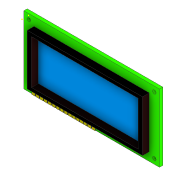
# Autodesk Inventor part: lcd display
Saved by Autodesk Inventor 2021 (Build 250183000, 183)
## iProperties
Created: 2021-06-25
Part Number: lcd display
Material: Generic
Document SubType Name: Modeling
Designer: Dell
Density: 1 g/cm^3
Appearance: Default
Author: Dell
Autodesk Inventor part; units mm, degrees
ref_plane "YZ Plane" through (0, 0, 0) normal (1, 0, 0) x (0, 1, 0)
ref_plane "XZ Plane" through (0, 0, 0) normal (0, 1, 0) x (-1, 0, 0)
sketch "Sketch2" plane through (0, 0, 0) normal (0, 0, 1) x (1, 0, 0)
  line L0 (-14.0665, 4.9582) -> (385.9335, 4.9582)
  line L1 (385.9335, 4.9582) -> (385.9335, -195.0418)
  line L2 (385.9335, -195.0418) -> (-14.0665, -195.0418)
  line L3 (-14.0665, -195.0418) -> (-14.0665, 4.9582)
  circle A0 centre (0.9335, -10.0418) radius 5
  circle A1 centre (370.9335, -10.0418) radius 5
  circle A2 centre (0.9335, -180.0418) radius 5
  circle A3 centre (370.9335, -180.0418) radius 5
  point P0 (0, 0)
  dimension "d3" = 400
  dimension "d4" = 200
  dimension "d5" = 10
  dimension "d6" = 10
  dimension "d7" = 10
  dimension "d8" = 10
  dimension "d9" = 15
  dimension "d10" = 15
  dimension "d11" = 15
  dimension "d12" = 15
  dimension "d13" = 15
  dimension "d14" = 15
  dimension "d15" = 15
  dimension "d16" = 15
  constraints: 8 end point, 4 centre point, 2 parallel, 1 horizontal, 1 perpendicular
  measures "d3" distance of L1.end L2.end
  measures "d4" distance of L0.end L1.end
  measures "d5" diameter of A0
  measures "d6" diameter of A1
  measures "d7" diameter of A2
  measures "d8" diameter of A3
  measures "d9" distance from line of L0 A0.centre
  measures "d10" distance from line of L3 A0.centre
  measures "d11" distance from line of L2 A2.centre
  measures "d12" distance from line of L3 A2.centre
  measures "d13" distance from line of L1 A1.centre
  measures "d14" distance from line of L0 A1.centre
  measures "d15" distance from line of L1 A3.centre
  measures "d16" distance from line of L2 A3.centre
extrude "Extrusion1" add sketch "Sketch2" along normal blind 10
sketch "Sketch3" plane through (0, 0, 10) normal (0, 0, 1) x (1, 0, 0)
  line L0 (15.9335, -20.0418) -> (355.9335, -20.0418)
  line L1 (355.9335, -20.0418) -> (355.9335, -170.0418)
  line L2 (355.9335, -170.0418) -> (15.9335, -170.0418)
  line L3 (15.9335, -170.0418) -> (15.9335, -20.0418)
  line L4 (385.9335, 4.9582) -> (-14.0665, 4.9582) projected
  line L5 (385.9335, -195.0418) -> (385.9335, 4.9582) projected
  point P0 (0, 0)
  dimension "d20" = 340
  dimension "d21" = 150
  dimension "d22" = 25
  dimension "d23" = 30
  constraints: 8 end point, 2 parallel, 1 horizontal, 1 perpendicular
  measures "d20" distance of L1.end L2.end
  measures "d21" distance of L0.end L1.end
  measures "d22" distance between parallel lines of L0 L4
  measures "d23" distance between parallel lines of L5 L1
extrude "Extrusion2" add sketch "Sketch3" along normal blind 20
sketch "Sketch4" plane through (0, 0, 30) normal (0, 0, 1) x (1, 0, 0)
  point P0 (0, 0)
sketch "Sketch5" plane through (0, 0, 30) normal (0, 0, 1) x (1, 0, 0)
  point P0 (0, 0)
sketch "Sketch6" plane through (0, 0, 30) normal (0, 0, 1) x (1, 0, 0)
  line L0 (-14.0665, -195.0418) -> (385.9335, -195.0418) projected
  line L1 (10.9169, -195.0418) -> (10.9169, -178.0418)
  line L2 (10.9169, -195.0418) -> (20.9169, -195.0418)
  line L3 (20.9169, -195.0418) -> (20.9169, -178.0418)
  arc A0 (20.9169, -178.0418) -> (10.9169, -178.0418) centre (15.9169, -178.0418) ccw
  line L4 (20.9169, -195.0418) -> (22.9169, -195.0418)
  line L5 (22.9169, -195.0418) -> (22.9169, -178.0418)
  line L6 (22.9169, -195.0418) -> (32.9169, -195.0418)
  line L7 (32.9169, -195.0418) -> (32.9169, -178.0418)
  arc A1 (32.9169, -178.0418) -> (22.9169, -178.0418) centre (27.9169, -178.0418) ccw
  line L8 (34.9169, -195.0418) -> (34.9169, -178.0418)
  line L9 (34.9169, -195.0418) -> (44.9169, -195.0418)
  line L10 (44.9169, -195.0418) -> (44.9169, -178.0418)
  arc A2 (44.9169, -178.0418) -> (34.9169, -178.0418) centre (39.9169, -178.0418) ccw
  line L11 (46.9169, -195.0418) -> (46.9169, -178.0418)
  line L12 (46.9169, -195.0418) -> (56.9169, -195.0418)
  line L13 (56.9169, -195.0418) -> (56.9169, -178.0418)
  arc A3 (56.9169, -178.0418) -> (46.9169, -178.0418) centre (51.9169, -178.0418) ccw
  line L14 (58.9169, -195.0418) -> (58.9169, -178.0418)
  line L15 (58.9169, -195.0418) -> (68.9169, -195.0418)
  line L16 (68.9169, -195.0418) -> (68.9169, -178.0418)
  arc A4 (68.9169, -178.0418) -> (58.9169, -178.0418) centre (63.9169, -178.0418) ccw
  line L17 (70.9169, -195.0418) -> (70.9169, -178.0418)
  line L18 (70.9169, -195.0418) -> (80.9169, -195.0418)
  line L19 (80.9169, -195.0418) -> (80.9169, -178.0418)
  arc A5 (80.9169, -178.0418) -> (70.9169, -178.0418) centre (75.9169, -178.0418) ccw
  line L20 (82.9169, -195.0418) -> (82.9169, -178.0418)
  line L21 (82.9169, -195.0418) -> (92.9169, -195.0418)
  line L22 (92.9169, -195.0418) -> (92.9169, -178.0418)
  arc A6 (92.9169, -178.0418) -> (82.9169, -178.0418) centre (87.9169, -178.0418) ccw
  line L23 (94.9169, -195.0418) -> (94.9169, -178.0418)
  line L24 (94.9169, -195.0418) -> (104.9169, -195.0418)
  line L25 (104.9169, -195.0418) -> (104.9169, -178.0418)
  arc A7 (104.9169, -178.0418) -> (94.9169, -178.0418) centre (99.9169, -178.0418) ccw
  line L26 (106.9169, -195.0418) -> (106.9169, -178.0418)
  line L27 (106.9169, -195.0418) -> (116.9169, -195.0418)
  line L28 (116.9169, -195.0418) -> (116.9169, -178.0418)
  arc A8 (116.9169, -178.0418) -> (106.9169, -178.0418) centre (111.9169, -178.0418) ccw
  line L29 (118.9169, -195.0418) -> (118.9169, -178.0418)
  line L30 (118.9169, -195.0418) -> (128.9169, -195.0418)
  line L31 (128.9169, -195.0418) -> (128.9169, -178.0418)
  arc A9 (128.9169, -178.0418) -> (118.9169, -178.0418) centre (123.9169, -178.0418) ccw
  line L32 (129.9169, -195.0418) -> (129.9169, -178.0418)
  line L33 (129.9169, -195.0418) -> (139.9169, -195.0418)
  line L34 (139.9169, -195.0418) -> (139.9169, -178.0418)
  arc A10 (139.9169, -178.0418) -> (129.9169, -178.0418) centre (134.9169, -178.0418) ccw
  line L35 (141.9169, -195.0418) -> (141.9169, -178.0418)
  line L36 (141.9169, -195.0418) -> (151.9169, -195.0418)
  line L37 (151.9169, -195.0418) -> (151.9169, -178.0418)
  arc A11 (151.9169, -178.0418) -> (141.9169, -178.0418) centre (146.9169, -178.0418) ccw
  line L38 (152.9169, -195.0418) -> (152.9169, -178.0418)
  line L39 (152.9169, -195.0418) -> (162.9169, -195.0418)
  line L40 (162.9169, -195.0418) -> (162.9169, -178.0418)
  arc A12 (162.9169, -178.0418) -> (152.9169, -178.0418) centre (157.9169, -178.0418) ccw
  line L41 (163.9169, -195.0418) -> (163.9169, -178.0418)
  line L42 (163.9169, -195.0418) -> (173.9169, -195.0418)
  line L43 (173.9169, -195.0418) -> (173.9169, -178.0418)
  arc A13 (173.9169, -178.0418) -> (163.9169, -178.0418) centre (168.9169, -178.0418) ccw
  line L44 (185.9169, -195.0418) -> (185.9169, -178.0418)
  line L45 (175.9169, -195.0418) -> (185.9169, -195.0418)
  line L46 (175.9169, -195.0418) -> (175.9169, -178.0418)
  arc A14 (185.9169, -178.0418) -> (175.9169, -178.0418) centre (180.9169, -178.0418) ccw
  line L47 (197.9169, -195.0418) -> (197.9169, -178.0418)
  line L48 (187.9169, -195.0418) -> (197.9169, -195.0418)
  line L49 (187.9169, -195.0418) -> (187.9169, -178.0418)
  arc A15 (197.9169, -178.0418) -> (187.9169, -178.0418) centre (192.9169, -178.0418) ccw
  line L50 (28.4335, -30.0418) -> (343.4335, -30.0418)
  line L51 (343.4335, -30.0418) -> (343.4335, -160.0418)
  line L52 (343.4335, -160.0418) -> (28.4335, -160.0418)
  line L53 (28.4335, -160.0418) -> (28.4335, -30.0418)
  line L54 (355.9335, -20.0418) -> (15.9335, -20.0418) projected
  line L55 (15.9335, -20.0418) -> (15.9335, -170.0418) projected
  point P0 (0, 0)
  dimension "d27" = 17
  dimension "d28" = 10
  dimension "d29" = 17
  dimension "d30" = 2
  dimension "d31" = 10
  dimension "d32" = 17
  dimension "d33" = 5
  dimension "d34" = 10
  dimension "d35" = 17
  dimension "d36" = 5
  dimension "d37" = 10
  dimension "d38" = 17
  dimension "d39" = 5
  dimension "d40" = 10
  dimension "d41" = 17
  dimension "d42" = 5
  dimension "d43" = 10
  dimension "d44" = 17
  dimension "d45" = 5
  dimension "d46" = 10
  dimension "d47" = 17
  dimension "d48" = 5
  dimension "d49" = 10
  dimension "d50" = 17
  dimension "d51" = 5
  dimension "d52" = 10
  dimension "d53" = 17
  dimension "d54" = 5
  dimension "d55" = 10
  dimension "d56" = 17
  dimension "d57" = 5
  dimension "d58" = 10
  dimension "d59" = 17
  dimension "d60" = 5
  dimension "d61" = 10
  dimension "d62" = 17
  dimension "d63" = 5
  dimension "d64" = 10
  dimension "d65" = 17
  dimension "d66" = 5
  dimension "d67" = 10
  dimension "d68" = 17
  dimension "d69" = 5
  dimension "d70" = 2
  dimension "d71" = 2
  dimension "d72" = 2
  dimension "d73" = 2
  dimension "d74" = 2
  dimension "d75" = 2
  dimension "d76" = 2
  dimension "d77" = 2
  dimension "d78" = 1
  dimension "d79" = 2
  dimension "d80" = 1
  dimension "d81" = 1
  dimension "d82" = 10
  dimension "d83" = 17
  dimension "d84" = 5
  dimension "d85" = 10
  dimension "d86" = 17
  dimension "d87" = 5
  dimension "d88" = 2
  dimension "d89" = 2
  dimension "d90" = 315
  constraints: 106 end point, 32 point on circle, 16 centre point, 3 vertical, 2 parallel, 2 perpendicular, 1 horizontal, 1 tangent, 5 other
  measures "d27" distance of L1.start L1.end
  measures "d28" distance of L1.start L2.end
  measures "d29" distance of L2.end L3.end
  measures "d30" distance of L2.end L4.end
  measures "d31" distance of L4.end L6.end
  measures "d32" distance of L6.end L7.end
  measures "d33" radius of A1
  measures "d34" distance of L9.start L10.start
  measures "d35" distance of L10.start L10.end
  measures "d36" radius of A2
  measures "d37" distance of L12.start L13.start
  measures "d38" distance of L13.start L13.end
  measures "d39" radius of A3
  measures "d40" distance of L15.start L16.start
  measures "d41" distance of L16.start L16.end
  measures "d42" radius of A4
  measures "d43" distance of L18.start L19.start
  measures "d44" distance of L19.start L19.end
  measures "d45" radius of A5
  measures "d46" distance of L21.start L22.start
  measures "d47" distance of L22.start L22.end
  measures "d48" radius of A6
  measures "d49" distance of L24.start L25.start
  measures "d50" distance of L25.start L25.end
  measures "d51" radius of A7
  measures "d52" distance of L27.start L28.start
  measures "d53" distance of L28.start L28.end
  measures "d54" radius of A8
  measures "d55" distance of L30.start L31.start
  measures "d56" distance of L31.start L31.end
  measures "d57" radius of A9
  measures "d58" distance of L33.start L34.start
  measures "d59" distance of L34.start L34.end
  measures "d60" radius of A10
  measures "d61" distance of L36.start L37.start
  measures "d62" distance of L37.start L37.end
  measures "d63" radius of A11
  measures "d64" distance of L39.start L40.start
  measures "d65" distance of L40.start L40.end
  measures "d66" radius of A12
  measures "d67" distance of L42.start L43.start
  measures "d68" distance of L43.start L43.end
  measures "d69" radius of A13
  measures "d70" distance between parallel lines of L8 L7
  measures "d71" distance between parallel lines of L11 L10
  measures "d72" distance between parallel lines of L14 L13
  measures "d73" distance between parallel lines of L17 L16
  measures "d74" distance between parallel lines of L20 L19
  measures "d75" distance between parallel lines of L23 L22
  measures "d76" distance between parallel lines of L26 L25
  measures "d77" distance between parallel lines of L29 L28
  measures "d78" distance from line of L31.start L32
  measures "d79" distance between parallel lines of L35 L34
  measures "d80" distance between parallel lines of L38 L37
  measures "d81" distance between parallel lines of L41 L40
  measures "d82" distance of L45.start L45.end
  measures "d83" distance of L45.end L44.end
  measures "d84" radius of A14
  measures "d85" distance of L48.start L48.end
  measures "d86" distance of L48.end L47.end
  measures "d87" radius of A15
  measures "d88" distance between parallel lines of L46 L43
  measures "d89" distance between parallel lines of L49 L44
  measures "d90" distance of L51.end L52.end
extrude "Extrusion3" add sketch "Sketch6" along normal blind 1 contours L1 A0 L3 L0 | L5 A1 L7 L0 | L8 A2 L10 L0 | L11 A3 L13 L0 | L14 A4 L16 L0 | L17 A5 L19 L0 | L20 A6 L22 L0 | L23 A7 L25 L0 | L26 A8 L28 L0 | L29 A9 L31 L0 | L32 A10 L34 L0 | L35 A11 L37 L0 | L38 A12 L40 L0 | L41 A13 L43 L0 | L46 A14 L44 L0 | L49 A15 L47 L0
sketch "Sketch7" plane through (0, 0, 30) normal (0, 0, 1) x (1, 0, 0)
  point P0 (0, 0)
sketch "Sketch8" plane through (0, 0, 30) normal (0, 0, 1) x (1, 0, 0)
  line L0 (28.4335, -30.0418) -> (343.4335, -30.0418)
  line L1 (343.4335, -30.0418) -> (343.4335, -160.0418)
  line L2 (343.4335, -160.0418) -> (28.4335, -160.0418)
  line L3 (28.4335, -160.0418) -> (28.4335, -30.0418)
  line L4 (355.9335, -20.0418) -> (15.9335, -20.0418) projected
  line L5 (15.9335, -20.0418) -> (15.9335, -170.0418) projected
  point P0 (0, 0)
  dimension "d96" = 315
  dimension "d97" = 130
  dimension "d98" = 10
  dimension "d99" = 12.5
  constraints: 8 end point, 2 parallel, 1 horizontal, 1 perpendicular
  measures "d96" distance of L1.end L2.end
  measures "d97" distance of L0.end L1.end
  measures "d98" distance between parallel lines of L0 L4
  measures "d99" distance between parallel lines of L5 L3
extrude "Extrusion4" cut sketch "Sketch8" against normal blind 20
sketch "Sketch9" plane through (0, 0, 10) normal (0, 0, 1) x (1, 0, 0)
  point P0 (0, 0)
sketch "Sketch10" plane through (0, 0, 10) normal (0, 0, 1) x (1, 0, 0)
  point P0 (0, 0)
sketch "Sketch11" plane through (0, 0, 10) normal (0, 0, 1) x (1, 0, 0)
  point P0 (0, 0)
sketch "Sketch12" plane through (0, 0, 10) normal (0, 0, 1) x (1, 0, 0)
  point P0 (0, 0)
ref_plane "Work Plane1" through (0, 0, 11) normal (0, 0, 1) x (1, 0, 0)
sketch "Sketch13" plane through (0, 0, 10) normal (0, 0, 1) x (1, 0, 0)
  point P0 (0, 0)
sketch "Sketch14" plane through (0, 0, 10) normal (0, 0, 1) x (1, 0, 0)
  point P0 (0, 0)
thicken "Thicken1" operation add thickness 20 both sides no extend neighbours no toward (0, 0, -1) faces at (14.2503, -183.7084, 31)
thicken "Thicken2" operation add thickness 20 both sides no extend neighbours no toward (0, 0, -1) faces at (26.2503, -183.7084, 31)
thicken "Thicken3" operation add thickness 20 both sides no extend neighbours no toward (0, 0, -1) faces at (41.5836, -183.7084, 31)
thicken "Thicken4" operation add thickness 20 both sides no extend neighbours no toward (0, 0, -1) faces at (53.5836, -183.7084, 31)
thicken "Thicken5" operation add thickness 20 both sides no extend neighbours no toward (0, 0, -1) faces at (65.5836, -183.7084, 31)
thicken "Thicken6" operation add thickness 20 both sides no extend neighbours no toward (0, 0, -1) faces at (74.2503, -189.3751, 31)
thicken "Thicken7" operation add thickness 20 both sides no extend neighbours no toward (0, 0, -1) faces at (86.2503, -189.3751, 31)
thicken "Thicken8" operation add thickness 20 both sides no extend neighbours no toward (0, 0, -1) faces at (98.2503, -189.3751, 31)
thicken "Thicken9" operation add thickness 20 both sides no extend neighbours no toward (0, 0, -1) faces at (110.2503, -189.3751, 31)
thicken "Thicken10" operation add thickness 20 both sides no extend neighbours no toward (0, 0, -1) faces at (122.2503, -189.3751, 31)
thicken "Thicken11" operation add thickness 20 both sides no extend neighbours no toward (0, 0, -1) faces at (133.2503, -183.7084, 31)
thicken "Thicken12" operation cut thickness 19 both sides no extend neighbours no toward (0, 0, -1) faces at (14.2503, -183.7084, 31)
thicken "Thicken13" operation add thickness 20 both sides no extend neighbours no toward (0, 0, -1) faces at (145.2503, -183.7084, 31)
thicken "Thicken14" operation add thickness 20 both sides no extend neighbours no toward (0, 0, -1) faces at (156.2503, -183.7084, 31)
thicken "Thicken15" operation add thickness 20 both sides no extend neighbours no toward (0, 0, -1) faces at (167.2503, -183.7084, 31)
thicken "Thicken16" operation add thickness 20 both sides no extend neighbours no toward (0, 0, -1) faces at (182.5836, -189.3751, 31)
thicken "Thicken17" operation add thickness 20 both sides no extend neighbours no toward (0, 0, -1) faces at (194.5836, -189.3751, 31)
thicken "Thicken18" operation cut thickness 19 both sides no extend neighbours no toward (0, 0, -1) faces at (26.2503, -183.7084, 31)
thicken "Thicken19" operation cut thickness 19 both sides no extend neighbours no toward (0, 0, -1) faces at (41.5836, -183.7084, 31)
thicken "Thicken20" operation cut thickness 19 both sides no extend neighbours no toward (0, 0, -1) faces at (53.5836, -183.7084, 31)
thicken "Thicken21" operation cut thickness 19 both sides no extend neighbours no toward (0, 0, -1) faces at (65.5836, -183.7084, 31)
thicken "Thicken22" operation cut thickness 19 both sides no extend neighbours no toward (0, 0, -1) faces at (74.2503, -189.3751, 31)
thicken "Thicken23" operation cut thickness 19 both sides no extend neighbours no toward (0, 0, -1) faces at (86.2503, -189.3751, 31)
thicken "Thicken24" operation cut thickness 19 both sides no extend neighbours no toward (0, 0, -1) faces at (98.2503, -189.3751, 31)
thicken "Thicken25" operation cut thickness 19 both sides no extend neighbours no toward (0, 0, -1) faces at (110.2503, -189.3751, 31)
thicken "Thicken26" operation cut thickness 19 both sides no extend neighbours no toward (0, 0, -1) faces at (122.2503, -189.3751, 31)
thicken "Thicken27" operation cut thickness 19 both sides no extend neighbours no toward (0, 0, -1) faces at (133.2503, -183.7084, 31)
thicken "Thicken28" operation cut thickness 19 both sides no extend neighbours no toward (0, 0, -1) faces at (145.2503, -183.7084, 31)
thicken "Thicken29" operation cut thickness 19 both sides no extend neighbours no toward (0, 0, -1) faces at (156.2503, -183.7084, 31)
thicken "Thicken30" operation cut thickness 19 both sides no extend neighbours no toward (0, 0, -1) faces at (167.2503, -183.7084, 31)
thicken "Thicken31" operation cut thickness 19 both sides no extend neighbours no toward (0, 0, -1) faces at (182.5836, -189.3751, 31)
thicken "Thicken32" operation cut thickness 19 both sides no extend neighbours no toward (0, 0, -1) faces at (194.5836, -189.3751, 31)
body "Solid1"
